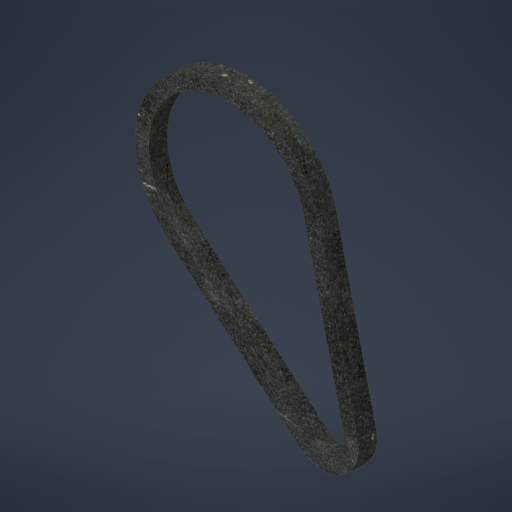
# Autodesk Inventor part: EL2-CGB-009
Saved by Autodesk Inventor 2023.4 (Build 274418000, 418)
## iProperties
Created: 2025-01-24
Part Number: EL2-CGB-009
Material: Steel
Document SubType Name: Modeling
Designer: brand
Density: 7.85 g/cm^3
Appearance: Plate
Author: brand
Autodesk Inventor part; units mm, degrees
ref_plane "YZ Plane" through (0, 0, 0) normal (1, 0, 0) x (0, 1, 0)
ref_plane "XZ Plane" through (0, 0, 0) normal (0, 1, 0) x (-1, 0, 0)
ref_plane "XY Plane" through (0, 0, 0) normal (0, 0, 1) x (1, 0, 0)
sketch "Sketch1" plane through (0, 0, 0) normal (0, 0, 1) x (1, 0, 0)
  circle A0 centre (0, 0) radius 18.1864 construction
  circle A1 centre (-61.1981, 101.1124) radius 54.5719 construction
  line L0 (-61.1981, 101.1124) -> (0, 0) construction
  arc A2 (-12.3694, 112.6139) -> (-94.0337, 63.1868) centre (-61.1981, 101.1124) ccw
  arc A3 (-9.0194, -10.4175) -> (13.4124, 3.1593) centre (0, 0) ccw
  line L1 (-94.0337, 63.1868) -> (-9.0194, -10.4175)
  line L2 (-12.3694, 112.6139) -> (13.4124, 3.1593)
  line L3 (-14.7885, -17.0809) -> (-99.8028, 56.5234)
  arc A4 (-3.7904, 114.6347) -> (-99.8028, 56.5234) centre (-61.1981, 101.1124) ccw
  line L4 (-3.7904, 114.6347) -> (21.9915, 5.1801)
  arc A5 (-14.7885, -17.0809) -> (21.9915, 5.1801) centre (0, 0) ccw
  line L5 (-11.9039, -13.7492) -> (-96.9182, 59.8551) construction
  arc A6 (-8.0799, 113.6243) -> (-96.9182, 59.8551) centre (-61.1981, 101.1124) ccw construction
  line L6 (-8.0799, 113.6243) -> (17.7019, 4.1697) construction
  arc A7 (-11.9039, -13.7492) -> (17.7019, 4.1697) centre (0, 0) ccw construction
  dimension "d0" = 36.3728
  dimension "d1" = 109.1438
  dimension "d2" = 118.1902
  dimension "d3" = 8.8138
  dimension "d4" = 61.1981
  dimension "d5" = 4.4069
  constraints: 14 end point, 12 point on circle, 8 centre point, 6 tangent, 2 coincident, 6 other
  measures "d0" diameter of A0
  measures "d1" diameter of A1
  measures "d2" distance of L0.start L0.end
  measures "d3" distance between parallel lines of L1 L3
  measures "d4" horizontal distance of L0.end L0.start
  measures "d5" distance between parallel lines of L1 L5
extrude "Extrusion1" add sketch "Sketch1" along normal mid plane 11.8364
equation "\"d5\" = 0.5 * d3"
body "Solid1"
